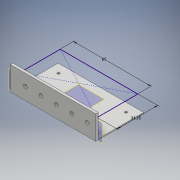
# Autodesk Inventor part: avhzy_maunt
Saved by Autodesk Inventor 2018 (Build 220112000, 112)
## iProperties
Created: 2019-07-20
Part Number: avhzy_maunt
Material: 一般
Document SubType Name: Modeling
Designer: guest1
Density: 1 g/cm^3
Appearance: 既定
Author: guest1
Autodesk Inventor part; units mm, degrees
ref_plane "YZ Plane" through (0, 0, 0) normal (1, 0, 0) x (0, 1, 0)
ref_plane "XZ Plane" through (0, 0, 0) normal (0, 1, 0) x (-1, 0, 0)
ref_plane "XY Plane" through (0, 0, 0) normal (0, 0, 1) x (1, 0, 0)
sketch "スケッチ1" plane through (0, 0, 0) normal (0, 0, 1) x (1, 0, 0)
  line L0 (-32.5, -17.075) -> (32.5, -17.075)
  line L1 (32.5, -17.075) -> (32.5, 17.075)
  line L2 (32.5, 17.075) -> (-32.5, 17.075)
  line L3 (-32.5, 17.075) -> (-32.5, -17.075)
  line L4 (-32.5, -17.075) -> (32.5, 17.075) construction
  line L5 (32.5, -17.075) -> (-32.5, 17.075) construction
  point P0 (0, 0)
  dimension "d0" = 65
  dimension "d1" = 34.15
  constraints: 12 end point, 2 midpoint, 2 parallel, 1 horizontal, 1 perpendicular
  measures "d0" distance of L1.end L2.end
  measures "d1" distance of L0.end L1.end
ref_plane "作業平面2" through (0, 0, -11.7) normal (0, 0, -1) x (-1, 0, 0)
ref_plane "作業平面1" through (35.75, -19.2175, -13.7) normal (0, 1, 0) x (-1, 0, 0)
sketch "スケッチ3" plane through (35.75, -19.2175, -13.7) normal (0, 1, 0) x (-1, 0, 0)
  line L0 (71.5, 0) -> (0, 0)
  line L1 (0, 0) -> (71.5, 0)
  line L2 (71.5, 0) -> (71.5, 20)
  line L3 (71.5, 20) -> (0, 20)
  line L4 (0, 20) -> (0, 0)
  line L5 (71.5, 1) -> (0, 1) projected
  point P0 (35.75, 13.7)
  dimension "d6" = 20
  dimension "d10" = 1
  constraints: 10 end point
  measures "d6" distance of L0.start L2.end
  measures "d10" distance between parallel lines of L5 L0
extrude "押し出し3" add sketch "スケッチ3" against normal blind 2
sketch "スケッチ4" plane through (35.75, -19.2175, -13.7) normal (0, 1, 0) x (1, 0, 0)
  line L0 (0, 0) -> (-71.5, 0) projected
  line L1 (0, -1) -> (-71.5, -1) projected
  line L2 (0, 0) -> (-71.5, 0)
  line L3 (-71.5, 0) -> (-71.5, -1)
  line L4 (-71.5, -1) -> (0, -1)
  line L5 (0, -1) -> (0, 0)
  point P0 (-35.75, -13.7)
  constraints: 8 end point, 2 parallel, 1 horizontal, 1 perpendicular
extrude "押し出し4" add sketch "スケッチ4" along normal blind 38
sketch "スケッチ5" plane through (35.75, -19.2175, -13.7) normal (0, 1, 0) x (1, 0, 0)
  line L0 (0, 0) -> (0, -20) projected
  line L1 (0, -10) -> (-71.5, -10.5)
  line L2 (-71.5, -1) -> (-71.5, -20) projected
  point P0 (-35.75, -13.7)
  point P1 (-7, -10.049)
  point P2 (-20, -10.1399)
  point P3 (-33, -10.2308)
  point P4 (-46, -10.3217)
  point P5 (-59, -10.4126)
  dimension "d13" = 71.5
  dimension "d14" = 7
  dimension "d15" = 13
  dimension "d16" = 13
  dimension "d17" = 13
  dimension "d18" = 13
  constraints: 5 point on line, 2 end point, 2 midpoint
  measures "d13" horizontal distance of L1.start L1.end
  measures "d14" horizontal distance of point (-7, -10.049) L1.start
  measures "d15" horizontal distance of point (-20, -10.14) point (-7, -10.049)
  measures "d16" horizontal distance of point (-20, -10.14) point (-33, -10.231)
  measures "d17" horizontal distance of point (-33, -10.231) point (-46, -10.322)
  measures "d18" horizontal distance of point (-59, -10.413) point (-46, -10.322)
hole "穴1" at (28.75, -19.2175, -3.651) at (15.75, -19.2175, -3.5601) at (2.75, -19.2175, -3.4692) at (-10.25, -19.2175, -3.3783) at (-23.25, -19.2175, -3.2874) direction (0, -1, 0) diameter 3 depth 2 tip angle 118
sketch "スケッチ6" plane through (35.75, -21.2175, -13.7) normal (0, 0, -1) x (-1, 0, 0)
  line L0 (0, 2) -> (0, 40) projected
  line L1 (0, 0) -> (71.5, 0) projected
  line L2 (0, 40) -> (71.5, 40) projected
  line L3 (64, 7.25) -> (7.5, 7.25)
  line L4 (7.5, 7.25) -> (7.5, 32.75)
  line L5 (7.5, 32.75) -> (64, 32.75)
  line L6 (64, 32.75) -> (64, 7.25)
  line L7 (64, 7.25) -> (7.5, 32.75) construction
  line L8 (7.5, 7.25) -> (64, 32.75) construction
  point P0 (35.75, 21.2175)
  point P1 (35.75, 20)
  dimension "d26" = 56.5
  dimension "d27" = 25.5
  constraints: 12 end point, 2 midpoint, 2 parallel, 1 horizontal, 1 perpendicular
  measures "d26" distance of L4.end L5.end
  measures "d27" distance of L3.end L4.end
hole "穴2" at (28.25, 11.5325, -13.7) at (28.25, -13.9675, -13.7) at (-28.25, 11.5325, -13.7) at (-28.25, -13.9675, -13.7) direction (0, 0, 1) diameter 2 depth 2 tip angle 118
